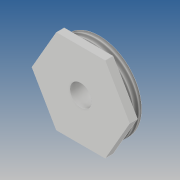
# Autodesk Inventor part: cartridge_locker_piston_top
Saved by Autodesk Inventor 2019 (Build 230136000, 136)
## iProperties
Created: 2019-03-17
Part Number: cartridge_locker_piston_top
Material: Générique
Document SubType Name: Modeling
Designer: Theo
Density: 1 g/cm^3
Appearance: Par défaut
Author: Theo
Autodesk Inventor part; units mm, degrees
ref_plane "YZ Plane" through (0, 0, 0) normal (1, 0, 0) x (0, 1, 0)
ref_plane "XZ Plane" through (0, 0, 0) normal (0, 1, 0) x (-1, 0, 0)
ref_plane "XY Plane" through (0, 0, 0) normal (0, 0, 1) x (1, 0, 0)
sketch "Esquisse1" plane through (0, 0, 0) normal (1, 0, 0) x (0, 1, 0)
  line L0 (0, 0) -> (0, -6.3939)
  line L1 (9.5, 0) -> (2.05, 0)
  line L2 (9.5, 0) -> (9.5, -1.5)
  line L3 (9.5, -1.5) -> (8, -1.5)
  line L4 (8, -1.5) -> (8, -3.5)
  line L5 (8, -3.5) -> (7, -3.5)
  line L6 (2.05, 0) -> (2.05, -3)
  line L7 (7, -3.5) -> (5.5, -3)
  line L8 (5.5, -3) -> (2.05, -3)
  dimension "d1" = 1.5
  dimension "d2" = 1.5
  dimension "d4" = 16
  dimension "d5" = 4.1
  dimension "d10" = 2
  dimension "d11" = 3
  dimension "d12" = 1.5
  dimension "d13" = 1
  constraints: 18 end point, 4 horizontal, 4 vertical, 1 horizontal alignment
  measures "d1" distance of L2.end L3.end
  measures "d2" distance of L1.start L2.end
  measures "d4" diameter of L4 L0
  measures "d5" diameter of L6 L0
  measures "d10" distance of L3.end L4.end
  measures "d11" distance of L1.end L6.end
  measures "d12" horizontal distance of L5.end L7.end
  measures "d13" distance of L4.end L5.end
revolve "Révolution1" add sketch "Esquisse1" angle 360 about axis through (0, 0, 0) along (0, 0, -1)
sketch "Esquisse2" plane through (0, 0, 0) normal (0, 0, 1) x (1, 0, 0)
  line L0 (4.6188, 8) -> (9.2376, 0)
  line L1 (9.2376, 0) -> (4.6188, -8)
  line L2 (4.6188, -8) -> (-4.6188, -8)
  line L3 (-4.6188, -8) -> (-9.2376, 0)
  line L4 (-9.2376, 0) -> (-4.6188, 8)
  line L5 (-4.6188, 8) -> (4.6188, 8)
  circle A0 centre (0, 0) radius 9.5 projected
  dimension "d7" = 16
  constraints: 12 end point, 1 coincident, 1 horizontal, 13 other
  measures "d7" distance between parallel lines of L2 L5
extrude "Extrusion1" cut sketch "Esquisse2" against normal up to surface (1.5 mm away)
thread "Filetage1" size "M16x1" class "6g" standard "ISO Metric profile" full length
